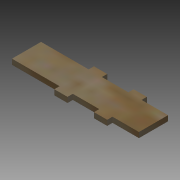
# Autodesk Inventor part: hlid
Saved by Autodesk Inventor 2016 (Build 200138000, 138)
## iProperties
Created: 2015-10-06
Part Number: hlid
Material: Generic
Document SubType Name: Modeling
Designer: Haukur
Density: 1 g/cm^3
Appearance: Plywood - Weathered
Author: Haukur
Autodesk Inventor part; units mm, degrees
ref_plane "YZ Plane" through (0, 0, 0) normal (1, 0, 0) x (0, 1, 0)
ref_plane "XZ Plane" through (0, 0, 0) normal (0, 1, 0) x (-1, 0, 0)
ref_plane "XY Plane" through (0, 0, 0) normal (0, 0, 1) x (1, 0, 0)
sketch "Sketch1" plane through (0, 0, 0) normal (0, 0, 1) x (1, 0, 0)
  line L0 (0, 4) -> (0, 26)
  line L1 (0, 26) -> (36, 26)
  line L2 (36, 26) -> (36, 30)
  line L3 (36, 30) -> (46, 30)
  line L4 (46, 30) -> (46, 26)
  line L5 (46, 26) -> (66, 26)
  line L6 (66, 26) -> (66, 30)
  line L7 (66, 30) -> (76, 30)
  line L8 (76, 30) -> (76, 26)
  line L9 (76, 26) -> (96, 26)
  line L10 (96, 26) -> (96, 4)
  line L11 (96, 4) -> (76, 4)
  line L12 (76, 4) -> (76, 0)
  line L13 (76, 0) -> (66, 0)
  line L14 (66, 0) -> (66, 4)
  line L15 (66, 4) -> (46, 4)
  line L16 (46, 4) -> (46, 0)
  line L17 (46, 0) -> (36, 0)
  line L18 (36, 4) -> (0, 4)
  line L19 (36, 0) -> (36, 4)
  point P0 (0, 0)
  dimension "d0" = 22
  dimension "d1" = 36
  dimension "d2" = 4
  dimension "d3" = 10
  dimension "d4" = 20
  dimension "d5" = 10
  dimension "d6" = 20
  constraints: 40 end point, 19 point on line, 11 perpendicular, 1 vertical
  measures "d0" distance of L0.start L0.end
  measures "d1" distance of L0.end L1.end
  measures "d2" distance of L1.end L2.end
  measures "d3" distance of L2.end L3.end
  measures "d4" distance of L4.end L5.end
  measures "d5" distance of L6.end L7.end
  measures "d6" distance of L8.end L9.end
extrude "Extrusion1" add sketch "Sketch1" along normal blind 4
body "Solid1"
